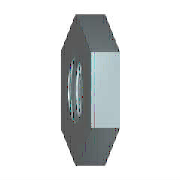
# Autodesk Inventor part: ISO 4036 - M2
Saved by Autodesk Inventor 2025.2 (Build 292293000, 293)
## iProperties
Created: 2024-01-20
Part Number: ISO 4036 - M2
Material: Steel
Description: Hexagon thin nuts(unchamfered) - product grade B
Document SubType Name: Modeling
Standard: ISO 4036
Designer: Kacper Mik
Standard Revision: Third edition 2012-12-15
Standards Organization: ISO
Language: en-US
Size Designation: M2
Categories: <MemberInstance><Categories><Category DisplayName="Fasteners" InternalName="e4da775c-781d-43d5-af7c-5136215cf5a6" Mnemonic="FSTN"><Category DisplayName="Nuts" InternalName="e37c7a56-0470-4688-8db4-b4d75d611516" Mnemonic="NUT"><CategoryParameter DisplayName="Thread Designation" InternalName="10aefdba-3783-44b8-becc-0feae870ab73" Mnemonic="thrdesign"/><CategoryParameter DisplayName="Thread Series Designation" InternalName="17a0ae10-6923-48a9-85c7-ae9b76790e6f" Mnemonic="thrserdsgn"/><CategoryParameter DisplayName="Thread Type" InternalName="205c6614-02f1-43b1-b704-b331415a8186" Mnemonic="thrtype"/><CategoryParameter DisplayName="Nominal Diameter Designation" InternalName="39406bc0-754a-4a9f-8c64-e1bba9d40b8a" Mnemonic="nomdiadesig"/><CategoryParameter DisplayName="Height" InternalName="5579c84d-d692-41f2-8996-171d03c19b53" Mnemonic="nheig"/><CategoryParameter DisplayName="Thread Class" InternalName="9b95427d-7bb5-461a-8a3e-4650073a592b" Mnemonic="thrclss"/><CategoryParameter DisplayName="Thread Pitch" InternalName="bd2c58b1-df6d-45e3-8bf7-4a0997b15b95" Mnemonic="pitch1"/><CategoryParameter DisplayName="Nominal Diameter" InternalName="d6e3b243-37ab-4432-98ea-592d296d3a46" Mnemonic="nomdia"/><CategoryParameter DisplayName="Threads per Unit" InternalName="e2e4d09d-bc7f-4af6-8086-8693b8d97bcd" Mnemonic="thrperunit1"/><Category DisplayName="Hex" InternalName="73d9c703-2233-4460-907f-38a87f245fbb" Mnemonic="PLNUT"><CategoryParameter DisplayName="Width Across Corners" InternalName="3db1d29f-9506-4e4b-a66f-416ec1d0915f" Mnemonic="wacor"/><CategoryParameter DisplayName="Type" InternalName="4e484966-9917-44a5-bcb5-b45bf8fff7e8" Mnemonic="type"/><CategoryParameter DisplayName="Property Class" InternalName="bcb84129-2a2e-4fb9-8398-d46bb849f471" Mnemonic="propclss"/></Category></Category></Category><Category DisplayName="DataType" InternalName="23b78d0f-2648-40c6-8793-ca6db495c9e8" Mnemonic="DATATYPE"><CategoryParameter DisplayName="DisplayName" InternalName="05415f3d-3907-474b-a020-eb9d644f4cf3" Mnemonic="DISPLAYNAME"/><CategoryParameter DisplayName="Standard" InternalName="0c0a119c-1e12-4c84-803f-101930972f5e" Mnemonic="STANDARD"/><CategoryParameter DisplayName="Description" InternalName="13903e3d-64b1-4950-80da-f627842ea37f" Mnemonic="DESCRIPTION"/><CategoryParameter DisplayName="Designation" InternalName="2675968c-4ce5-49e0-a4f5-552d29089031" Mnemonic="DESIGNATION"/><CategoryParameter DisplayName="Default Row" InternalName="2af9ec52-faaa-4026-b378-f9fa4afca842" Mnemonic="DEFAULTROW"/><CategoryParameter DisplayName="Folder Name" InternalName="3f06958e-8713-4116-9be7-ed6184ecc97b" Mnemonic="FOLDERNAME"/><CategoryParameter DisplayName="Revision Guid" InternalName="45a75005-10b1-4dfc-8d6d-dfe629f0b93c" Mnemonic="REVISIONGUID"/><CategoryParameter DisplayName="FileName" InternalName="8b46a4cc-9585-4fed-90c3-899f57e09a73" Mnemonic="FILENAME"/><CategoryParameter DisplayName="StdsOrg" InternalName="8f5914e1-4693-403f-8ab5-d37768198c9d" Mnemonic="STDSORG"/><CategoryParameter DisplayName="Family Version" InternalName="914462f6-6e19-4b14-ba84-155b9680b1d0" Mnemonic="FAMILYREVISION"/><CategoryParameter DisplayName="Standard Revision" InternalName="91d5a463-65c2-4fde-b823-3b7fea5e8e17" Mnemonic="STANDARDREVISION"/><CategoryParameter DisplayName="Member Revision" InternalName="a65d44b9-392f-4f4f-857b-e4b3d54996fe" Mnemonic="MEMBERREVISION"/><CategoryParameter DisplayName="ClipFormat" InternalName="bc51e27b-3422-4e78-93ef-cec197ddf230" Mnemonic="CLIPFORMAT"/><CategoryParameter DisplayName="Manufacturer" InternalName="cd6c7a72-a28a-4e50-99a9-2c7f4e13e5ad" Mnemonic="MANUFACTURER"/><CategoryParameter DisplayName="InternalName" InternalName="cf1d0246-76d9-4b4a-8305-fa0409afb5c1" Mnemonic="INTERNALNAME"/><CategoryParameter DisplayName="IsMetric" InternalName="e2385c5b-1ea4-4823-96a8-8de651266ec3" Mnemonic="ISMETRIC"/><Category DisplayName="Part" InternalName="c0e0b642-3bcb-4cc8-9e80-f96d35c4afa4" Mnemonic="PART"><CategoryParameter DisplayName="Part Number" InternalName="016b6077-bfbe-49bd-92c9-d8d59c39c941" Mnemonic="PARTNUMBER"/><CategoryParameter DisplayName="Stock Number" InternalName="4dba7c1c-e26c-444e-836c-b08b433409a8" Mnemonic="STOCKNUMBER"/><CategoryParameter DisplayName="Material Key" InternalName="5c9a8adb-dd2b-4535-b97f-0a94a95fe41f" Mnemonic="MATERIALKEY"/><CategoryParameter DisplayName="Material" InternalName="818a152a-d3c3-49ca-80ee-df7d91421b8e" Mnemonic="MATERIAL"/></Category></Category><Category DisplayName="Legacy Map DA" InternalName="924fff40-ddd0-4eff-ad42-30e3774ef79e" Mnemonic="LEGACYMAPDA"><CategoryParameter DisplayName="DACookie" InternalName="316934ee-8fe1-4c7a-9c36-f2d79e1add1a" Mnemonic="DACOOKIE"/></Category></Categories><FamilyTemplate Id="I4036"><FamilyTemplateParameters><FamilyTemplateParameter ObjectType="kUserParameterObject" ValueType="xs:double" Id="1" ObjectReferenceKey="NND"/><FamilyTemplateParameter ObjectType="kUserParameterObject" ValueType="xs:double" Id="2" ObjectReferenceKey="PTC"/><FamilyTemplateParameter ObjectType="kUserParameterObject" ValueType="xs:double" Id="3" ObjectReferenceKey="ParS"/><FamilyTemplateParameter ObjectType="kUserParameterObject" ValueType="xs:double" Id="4" ObjectReferenceKey="M"/><FamilyTemplateParameter ObjectType="kUserParameterObject" ValueType="xs:double" Id="116" ObjectReferenceKey="THREADDIA"/><FamilyTemplateParameter ObjectType="kPropertyObject" ValueType="xs:string" Id="100" ObjectReferenceKey="{32853F0F-3444-11d1-9E93-0060B03C1CA6}" SubObjectId="52"/><FamilyTemplateParameter ObjectType="kPropertyObject" ValueType="xs:string" Id="105" ObjectReferenceKey="{32853F0F-3444-11d1-9E93-0060B03C1CA6}" SubObjectId="5"/><FamilyTemplateParameter ObjectType="kPartComponentDefinitionObject" ValueType="xs:string" Id="110" SubObjectId="Material"/><FamilyTemplateParameter ObjectType="kThreadFeatureObject" ValueType="xs:structure" Id="300" ObjectReferenceKey="100200001000000017010000000000008000000000000000" SubObjectId="ThreadInfo"><FamilyTemplateParameter ObjectType="" ValueType="xs:string" Id="301" SubObjectId="ThreadDesignation"/><FamilyTemplateParameter ObjectType="" ValueType="xs:string" Id="302" SubObjectId="ThreadType"/><FamilyTemplateParameter ObjectType="" ValueType="xs:string" Id="303" SubObjectId="ThreadClass"/></FamilyTemplateParameter></FamilyTemplateParameters></FamilyTemplate><CategoryParameterMap><ParamToTemplateMap><ParamToTemplate CategoryParameter="//CategoryParameter[@InternalName='05415f3d-3907-474b-a020-eb9d644f4cf3']" ConstantValue="ISO 4036"/><ParamToTemplate CategoryParameter="//CategoryParameter[@InternalName='cf1d0246-76d9-4b4a-8305-fa0409afb5c1']" ConstantValue="4BE25EC3-BA07-4893-B857-6C8AA65813D5"/><ParamToTemplate CategoryParameter="//CategoryParameter[@InternalName='3f06958e-8713-4116-9be7-ed6184ecc97b']" ConstantValue="ISO 4036(2)"/><ParamToTemplate CategoryParameter="//CategoryParameter[@InternalName='914462f6-6e19-4b14-ba84-155b9680b1d0']" ConstantValue="10"/><ParamToTemplate CategoryParameter="//CategoryParameter[@InternalName='bc51e27b-3422-4e78-93ef-cec197ddf230']" ConstantValue="CF_INVENTOR.STDPARTS"/><ParamToTemplate CategoryParameter="//CategoryParameter[@InternalName='e2385c5b-1ea4-4823-96a8-8de651266ec3']" ConstantValue="true"/><ParamToTemplate CategoryParameter="//CategoryParameter[@InternalName='13903e3d-64b1-4950-80da-f627842ea37f']" ConstantValue="Hexagon thin nuts(unchamfered) - product grade B"/><ParamToTemplate CategoryParameter="//CategoryParameter[@InternalName='8f5914e1-4693-403f-8ab5-d37768198c9d']" ConstantValue="ISO"/><ParamToTemplate CategoryParameter="//CategoryParameter[@InternalName='0c0a119c-1e12-4c84-803f-101930972f5e']" ConstantValue="ISO 4036"/><ParamToTemplate CategoryParameter="//CategoryParameter[@InternalName='cd6c7a72-a28a-4e50-99a9-2c7f4e13e5ad']" TemplateParameter="104"/><ParamToTemplate CategoryParameter="//CategoryParameter[@InternalName='91d5a463-65c2-4fde-b823-3b7fea5e8e17']" ConstantValue="Third edition 2012-12-15"/><ParamToTemplate CategoryParameter="//CategoryParameter[@InternalName='45a75005-10b1-4dfc-8d6d-dfe629f0b93c']" ConstantValue="d8a7ba54-de08-41d3-9dcd-d5a2c9622f77"/><ParamToTemplate CategoryParameter="//CategoryParameter[@InternalName='2af9ec52-faaa-4026-b378-f9fa4afca842']" ConstantValue="10"/><ParamToTemplate CategoryParameter="//CategoryParameter[@InternalName='8b46a4cc-9585-4fed-90c3-899f57e09a73']" ConstantValue="ISO 4036 - M2(2)"/><ParamToTemplate CategoryParameter="//CategoryParameter[@InternalName='a65d44b9-392f-4f4f-857b-e4b3d54996fe']" ConstantValue="A20F2840-DB92-47A5-915C-9C0644CB75FF"/><ParamToTemplate CategoryParameter="//CategoryParameter[@InternalName='3db1d29f-9506-4e4b-a66f-416ec1d0915f']" ConstantValue="4,5712"/><ParamToTemplate CategoryParameter="//CategoryParameter[@InternalName='316934ee-8fe1-4c7a-9c36-f2d79e1add1a']" ConstantValue="*ISO~I4036~M2*"/><ParamToTemplate CategoryParameter="//CategoryParameter[@InternalName='2675968c-4ce5-49e0-a4f5-552d29089031']" TemplateParameter="100"/><ParamToTemplate CategoryParameter="//CategoryParameter[@InternalName='5579c84d-d692-41f2-8996-171d03c19b53']" TemplateParameter="4"/><ParamToTemplate CategoryParameter="//CategoryParameter[@InternalName='818a152a-d3c3-49ca-80ee-df7d91421b8e']" TemplateParameter="110"/><ParamToTemplate CategoryParameter="//CategoryParameter[@InternalName='d6e3b243-37ab-4432-98ea-592d296d3a46']" TemplateParameter="1"/><ParamToTemplate CategoryParameter="//CategoryParameter[@InternalName='016b6077-bfbe-49bd-92c9-d8d59c39c941']" TemplateParameter="105"/><ParamToTemplate CategoryParameter="//CategoryParameter[@InternalName='bd2c58b1-df6d-45e3-8bf7-4a0997b15b95']" TemplateParameter="2"/><ParamToTemplate CategoryParameter="//CategoryParameter[@InternalName='9b95427d-7bb5-461a-8a3e-4650073a592b']" TemplateParameter="303"/><ParamToTemplate CategoryParameter="//CategoryParameter[@InternalName='10aefdba-3783-44b8-becc-0feae870ab73']" TemplateParameter="301"/><ParamToTemplate CategoryParameter="//CategoryParameter[@InternalName='205c6614-02f1-43b1-b704-b331415a8186']" TemplateParameter="302"/></ParamToTemplateMap></CategoryParameterMap></MemberInstance>
Density: 7.85 g/cm^3
Appearance: Plate
IsCustomPart: 0
Author: Kacper Mik
Autodesk Inventor part; units mm, degrees
sketch "Sketch1" plane through (0, 0, 0) normal (0, 0, 1) x (1, 0, 0)
  circle A0 centre (0, 0) radius 2 construction
  line L0 (-2, 1.1547) -> (-2, -1.1547)
  line L1 (-2, -1.1547) -> (0, -2.3094)
  line L2 (0, -2.3094) -> (2, -1.1547)
  line L3 (2, -1.1547) -> (2, 1.1547)
  line L4 (2, 1.1547) -> (0, 2.3094)
  line L5 (0, 2.3094) -> (-2, 1.1547)
  line L6 (0, 3.2332) -> (0, -3.2332) projected
  line L7 (-2.8, 0) -> (2.8, 0) projected
  point P0 (0, 0)
  dimension "ParS" = 4
  constraints: 12 end point, 5 equal length, 5 tangent, 2 midpoint, 1 centre point, 1 parallel, 1 vertical
  measures "ParS" diameter of A0
extrude "Extrusion1" add sketch "Sketch1" along normal blind 1.2
sketch "Sketch2" plane through (0, 0, 1.2) normal (0, 0, 1) x (1, 0, 0)
  point P0 (0, 0)
  point P1 (0, 0)
  constraints: 1 coincident
hole "Hole1" at (0, 0, 1.2) direction (0, 0, -1) diameter 1.567 end through all thread size "M2x0.4" class "6H" standard "ISO Metric profile"
ref_plane "MSC_PT1" through (0, 0, 1.2) normal (0, 0, 1) x (1, 0, 0)
ref_plane "MSC_PT2" through (0, 0, 0) normal (0, 0, -1) x (-1, 0, 0)
ref_plane "MSC_PF1" through (0, 0, 0) normal (1, 0, 0) x (0, 1, 0)
chamfer "Chamfer1" distance 0.24 angle 45 2 edges at (0, 0.7835, 1.2) (0, 0.7835, 0)
equation "\"d17\" = 0.6 * PTC"
equation "\"d18\" = 0.6 * PTC"
equation "\"d4\" = M"
equation "\"PTC\" = 0.4"
equation "\"NND\" = 2"
equation "\"THREADDIA\" = NND"
body "Solid1"
